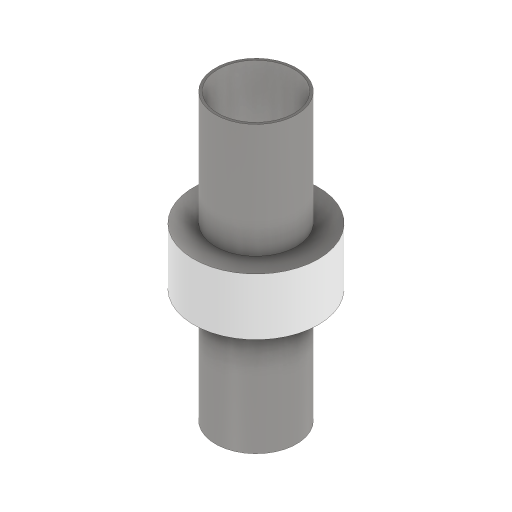
# Autodesk Inventor part: ICF34_Ceramic
Saved by Autodesk Inventor 2024.2 (Build 282272000, 272)
## iProperties
Created: 2022-11-25
Part Number: ICF34_Ceramic
Material: Stainless Steel, 440C
Document SubType Name: Modeling
Designer: kuzmin
Density: 7.75 g/cm^3
Appearance: Semi-Polished
Author: kuzmin
Autodesk Inventor part; units mm, degrees
ref_plane "YZ Plane" through (0, 0, 0) normal (1, 0, 0) x (0, 1, 0)
ref_plane "XZ Plane" through (0, 0, 0) normal (0, 1, 0) x (-1, 0, 0)
ref_plane "XY Plane" through (0, 0, 0) normal (0, 0, 1) x (1, 0, 0)
sketch "Sketch1" plane through (0, 0, 0) normal (0, 1, 0) x (-1, 0, 0)
  circle A0 centre (0, 0) radius 7.7
  circle A1 centre (0, 0) radius 8.2
  dimension "d0" = 15.4
  dimension "d1" = 16.4
  constraints: 2 centre point, 2 coincident
  measures "d0" diameter of A0
  measures "d1" diameter of A1
extrude "Extrusion1" add sketch "Sketch1" along normal blind 23.0816
sketch "Sketch2" plane through (0, 23.0816, 0) normal (0, 1, 0) x (1, 0, 0)
  circle A0 centre (0, 0) radius 12.6
  circle A1 centre (0, 0) radius 7.7 projected
  dimension "d4" = 25.2
  constraints: 1 centre point, 1 coincident
  measures "d4" diameter of A0
extrude "Extrusion2" add sketch "Sketch2" along normal blind 11.5
sketch "Sketch3" plane through (0, 34.5816, 0) normal (0, 1, 0) x (1, 0, 0)
  circle A0 centre (0, 0) radius 8.2 projected
  circle A1 centre (0, 0) radius 7.7 projected
extrude "Extrusion3" add sketch "Sketch3" along normal blind 23.0816
equation "\"delta\" = 7.0816"
body "Solid1"
